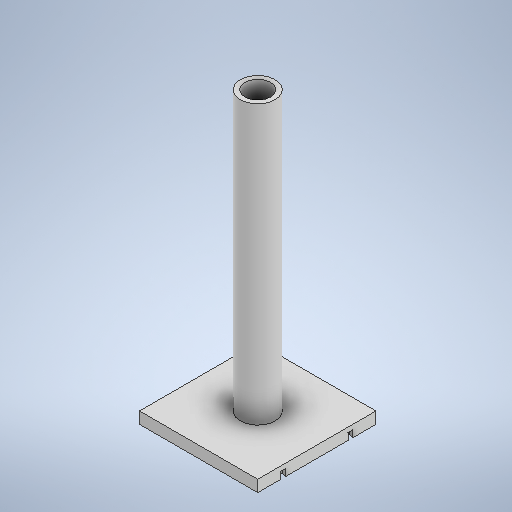
# Autodesk Inventor part: desoldering_wick_stand
Saved by Autodesk Inventor 2025.1 (Build 291241000, 241)
## iProperties
Created: 2024-10-24
Part Number: desoldering_wick_stand
Material: Generic
Document SubType Name: Modeling
Designer: kamil
Density: 1 g/cm^3
Appearance: Default
Author: kamil
Autodesk Inventor part; units mm, degrees
ref_plane "YZ Plane" through (0, 0, 0) normal (1, 0, 0) x (0, 1, 0)
ref_plane "XZ Plane" through (0, 0, 0) normal (0, 1, 0) x (-1, 0, 0)
ref_plane "XY Plane" through (0, 0, 0) normal (0, 0, 1) x (1, 0, 0)
sketch "Sketch1" plane through (0, 0, 0) normal (0, 1, 0) x (-1, 0, 0)
  line L0 (25.5, -25.5) -> (-25.5, -25.5)
  line L1 (-25.5, -25.5) -> (-25.5, 25.5)
  line L2 (-25.5, 25.5) -> (25.5, 25.5)
  line L3 (25.5, 25.5) -> (25.5, -25.5)
  line L4 (25.5, -25.5) -> (-25.5, 25.5) construction
  line L5 (-25.5, -25.5) -> (25.5, 25.5) construction
  point P0 (0, 0)
  dimension "d0" = 51
  dimension "d1" = 51
  constraints: 12 end point, 2 midpoint, 2 parallel, 1 horizontal, 1 perpendicular
  measures "d0" distance of L1.end L2.end
  measures "d1" distance of L0.end L1.end
extrude "Extrusion1" add sketch "Sketch1" along normal blind 5
sketch "Sketch2" plane through (0, 5, 0) normal (0, 1, 0) x (1, 0, 0)
  circle A0 centre (0, 0) radius 7.5
  dimension "d4" = 15
  constraints: 1 centre point, 1 coincident
  measures "d4" diameter of A0
extrude "Extrusion2" add sketch "Sketch2" along normal blind 120
sketch "Sketch3" plane through (0, 125, 0) normal (0, 1, 0) x (1, 0, 0)
  circle A0 centre (0, 0) radius 5.5
  dimension "d7" = 11
  constraints: 1 centre point, 1 coincident
  measures "d7" diameter of A0
extrude "Extrusion3" cut sketch "Sketch3" against normal blind 125
sketch "Sketch4" plane through (0, 0, 0) normal (0, -1, 0) x (1, 0, 0)
  line L0 (-25.5, -25.5) -> (-25.5, 25.5)
  line L1 (-25.5, 15.5) -> (-27.000887, 15.99867)
  line L2 (-27.000887, 15.99867) -> (-27.000887, 12.99867)
  line L3 (-27.000887, 12.99867) -> (-25.500887, 13.5)
  line L4 (-25.500887, 13.5) -> (-25.500887, 16.5)
  line L5 (-25.500887, 16.5) -> (-25.500887, 12.844087)
  line L6 (-25.5, -15.5) -> (-27, -16)
  line L7 (-27, -16) -> (-27, -13)
  line L8 (-27, -13) -> (-25.5, -13.5)
  line L9 (-25.5, -15.5) -> (-25.5, -13.5)
  line L10 (-25.5, -25.5) -> (-25.5, 25.5)
  point P0 (0, 0)
  point P1 (-25.500887, 15)
  point P2 (-25.500887, 15.500295)
  dimension "d10" = 3
  dimension "d11" = 3
  dimension "d12" = 2
  dimension "d13" = 1.5
  dimension "d14" = 10
  dimension "d15" = 3
  dimension "d16" = 2
  dimension "d17" = 1.5
  dimension "d18" = 10
  dimension "d19" = 1.5
  constraints: 18 end point, 4 point on line, 3 parallel, 2 equal length, 1 collinear, 1 midpoint, 1 vertical
  measures "d10" distance of L3.end L4.end
  measures "d11" distance of L1.end L2.end
  measures "d12" distance of L1.start L3.end
  measures "d13" distance from line of L2 point (-25.501, 15)
  measures "d14" distance of L0.end L1.start
  measures "d15" distance of L6.end L7.end
  measures "d16" distance of L8.end L6.start
  measures "d17" horizontal distance of L6.end L6.start
  measures "d18" distance of L0.start L6.start
  measures "d19" horizontal distance of L2.end L3.end
sketch "Sketch4 outline for Extrusion4" plane through (0, 0, 0) normal (0, -1, 0) x (1, 0, 0)
  line L0 (-27.000887, 15.99867) -> (-27.000887, 12.99867)
  line L1 (-25.500887, 15.500295) -> (-27.000887, 15.99867)
  line L2 (-25.500887, 13.5) -> (-25.500887, 15.500295)
  line L3 (-27.000887, 12.99867) -> (-25.500887, 13.5)
  line L4 (-27, -13) -> (-27, -16)
  line L5 (-25.5, -13.5) -> (-27, -13)
  line L6 (-25.5, -15.5) -> (-25.5, -13.5)
  line L7 (-27, -16) -> (-25.5, -15.5)
extrude "Extrusion4" add sketch "Sketch4 outline for Extrusion4" against normal blind 3
sketch "Sketch5" plane through (0, 0, 0) normal (0, -1, 0) x (1, 0, 0)
  line L0 (25.5, 25.5) -> (25.5, -25.5)
  line L1 (25.5, -15.5) -> (23.539279, -16)
  line L2 (23.539279, -16) -> (23.539279, -13)
  line L3 (23.539279, -13) -> (25.5, -13.5)
  line L4 (25.5, -15.5) -> (25.5, -13.5)
  line L5 (25.5, 15.5) -> (23.538534, 16)
  line L6 (23.538534, 16) -> (23.538534, 13)
  line L7 (23.538534, 13) -> (25.5, 13.5)
  line L8 (25.5, 15.5) -> (25.5, 13.5)
  point P0 (0, 0)
  dimension "d22" = 3
  dimension "d23" = 2
  dimension "d24" = 10
  dimension "d25" = 2
  dimension "d26" = 3
  dimension "d27" = 10
  constraints: 16 end point, 4 point on line, 3 parallel, 2 equal length, 1 vertical
  measures "d22" distance of L1.end L2.end
  measures "d23" distance of L3.end L1.start
  measures "d24" distance of L1.start L0.end
  measures "d25" distance of L5.start L7.end
  measures "d26" distance of L5.end L6.end
  measures "d27" distance of L5.start L0.start
extrude "Extrusion5" cut sketch "Sketch5" against normal blind 3
body "Solid1"
